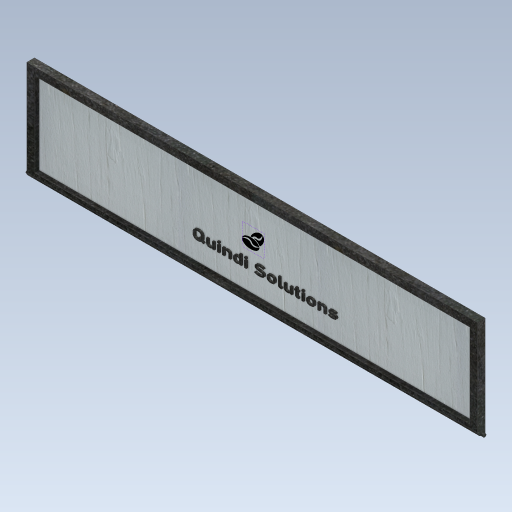
# Autodesk Inventor part: puerta
Saved by Autodesk Inventor 2023 (Build 270158000, 158)
## iProperties
Created: 2023-03-08
Part Number: puerta
Material: Steel
Document SubType Name: Modeling
Designer: santi
Density: 7.85 g/cm^3
Appearance: Plate
Author: santi
Autodesk Inventor part; units mm, degrees
ref_plane "YZ Plane" through (0, 0, 0) normal (1, 0, 0) x (0, 1, 0)
ref_plane "XZ Plane" through (0, 0, 0) normal (0, 1, 0) x (-1, 0, 0)
sketch "Sketch1" plane through (0, 0, 0) normal (0, 0, 1) x (1, 0, 0)
  line L0 (0, 0) -> (290, 0)
  line L1 (290, 0) -> (290, 64.12)
  line L2 (290, 64.12) -> (0, 64.12)
  line L3 (0, 64.12) -> (0, 0)
  line L4 (5, 59.12) -> (285, 59.12)
  line L5 (285, 59.12) -> (285, 5)
  line L6 (285, 5) -> (5, 5)
  line L7 (5, 5) -> (5, 59.12)
  dimension "d0" = 290
  dimension "d1" = 64.12
  dimension "d2" = 5
  constraints: 16 end point, 4 parallel, 2 perpendicular, 1 horizontal, 3 other
  measures "d0" distance of L2.end L1.end
  measures "d1" distance of L1.end L0.end
  measures "d2" distance between parallel lines of L2 L4
extrude "Extrusion1" add sketch "Sketch1" along normal blind 5
sketch "Sketch2" plane through (5, 5, 0) normal (1, 0, 0) x (0, 0, -1)
  line L0 (0, 54.12) -> (0, 0) projected
  line L1 (0, 54.12) -> (-5, 54.12) projected
  line L2 (0, 0) -> (-2, 0)
  line L3 (-2, 0) -> (-2, 54.12)
  line L4 (-2, 54.12) -> (0, 54.12)
  line L5 (0, 54.12) -> (0, 0)
  point P0 (0, -5)
  dimension "d5" = 2
  constraints: 8 end point, 2 parallel, 1 horizontal, 1 perpendicular, 1 point on line
  measures "d5" distance of L3.end L4.end
extrude "Extrusion2" add sketch "Sketch2" along normal up to surface (280 mm away)
sketch "Sketch3" plane through (0, 0, 0) normal (-1, 0, 0) x (0, 0, 1)
  circle A0 centre (2.5, 1) radius 1
  line L0 (5, 64.12) -> (5, 0) construction
  line L1 (0, 0) -> (5, 0) construction
  point P0 (2.5, 0)
  dimension "d8" = 2
  constraints: 1 centre point, 1 midpoint, 1 tangent, 1 vertical alignment
  measures "d8" diameter of A0
extrude "Extrusion3" add sketch "Sketch3" along normal blind 2 and the other way blind 2
ref_plane "Work Plane1" through (145, 0, 0) normal (1, 0, 0) x (0, 0, -1)
mirror "Mirror1" about plane through (145, 0, 0) normal (1, 0, 0) of "Extrusion3"
fillet "Fillet1" radius 2.7 1 edges at (145, 0, 5)
sketch "Sketch4" plane through (5, 5, 2) normal (0, 0, 1) x (1, 0, 0)
  line L0 (41.8121, 18.9) -> (199.4693, 18.9) construction
  line L1 (199.4693, 18.9) -> (199.4693, 1.1319) construction
  line L2 (199.4693, 1.1319) -> (41.8121, 1.1319) construction
  line L3 (41.8121, 1.1319) -> (41.8121, 18.9) construction
  line L4 (131.499, 39.7705) -> (150.9594, 39.7705) construction
  line L5 (150.9594, 39.7705) -> (150.9594, 20.3102) construction
  line L6 (150.9594, 20.3102) -> (131.499, 20.3102) construction
  line L7 (131.499, 20.3102) -> (131.499, 39.7705) construction
  spline S0 degree 2 poles (103.1114, 12.6741) (102.1443, 12.6741) (100.6936, 13.2282) (99.8927, 14.2457) (99.8927, 14.9207) knots 0 0 0 1 2 3 3 3
  line L8 (99.8927, 14.9207) -> (99.8927, 16.6484)
  spline S1 degree 2 poles (99.8927, 16.6484) (99.8927, 17.3284) (100.6936, 18.3409) (102.1443, 18.9) (103.1114, 18.9) knots 0 0 0 1 2 3 3 3
  spline S2 degree 2 poles (103.1114, 18.9) (104.0836, 18.9) (105.5292, 18.3409) (106.3302, 17.3284) (106.3302, 16.6484) knots 0 0 0 1 2 3 3 3
  line L9 (106.3302, 16.6484) -> (106.3302, 14.9207)
  spline S3 degree 2 poles (106.3302, 14.9207) (106.3302, 14.2457) (105.5292, 13.2282) (104.0836, 12.6741) (103.1114, 12.6741) knots 0 0 0 1 2 3 3 3
  spline S4 degree 2 poles (103.1114, 13.5153) (103.9728, 13.5153) (105.0155, 14.2709) (105.0155, 14.8904) knots 0 0 0 1 2 2 2
  line L10 (105.0155, 14.8904) -> (105.0155, 16.6786)
  spline S5 degree 2 poles (105.0155, 16.6786) (105.0155, 17.3032) (103.9728, 18.0538) (103.1114, 18.0538) knots 0 0 0 1 2 2 2
  spline S6 degree 2 poles (103.1114, 18.0538) (102.2551, 18.0538) (101.2124, 17.3032) (101.2124, 16.6786) knots 0 0 0 1 2 2 2
  line L11 (101.2124, 16.6786) -> (101.2124, 14.8904)
  spline S7 degree 2 poles (101.2124, 14.8904) (101.2124, 14.2709) (102.2551, 13.5153) (103.1114, 13.5153) knots 0 0 0 1 2 2 2
  line L12 (106.5065, 12.6338) -> (103.0913, 14.427)
  line L13 (103.0913, 14.427) -> (103.7612, 14.9912)
  line L14 (103.7612, 14.9912) -> (107.1714, 13.203)
  line L15 (107.1714, 13.203) -> (106.5065, 12.6338)
  line L16 (109.7151, 17.0917) -> (109.7151, 14.4421)
  spline S8 degree 2 poles (109.7151, 14.4421) (109.7151, 13.9837) (110.4153, 13.4851) (111.05, 13.4851) knots 0 0 0 1 2 2 2
  spline S9 degree 2 poles (111.05, 13.4851) (111.6847, 13.4851) (112.3697, 13.9334) (112.3697, 14.3414) knots 0 0 0 1 2 2 2
  line L17 (112.3697, 14.3414) -> (112.4604, 13.4297)
  spline S10 degree 2 poles (112.4604, 13.4297) (112.2841, 13.1375) (111.4026, 12.6741) (110.6923, 12.6741) knots 0 0 0 1 2 2 2
  spline S11 degree 2 poles (110.6923, 12.6741) (109.6093, 12.6741) (108.4306, 13.6009) (108.4306, 14.4421) knots 0 0 0 1 2 2 2
  line L18 (108.4306, 14.4421) -> (108.4306, 17.0917)
  line L19 (108.4306, 17.0917) -> (109.7151, 17.0917)
  line L20 (112.3697, 12.7345) -> (112.3697, 17.0917)
  line L21 (112.3697, 17.0917) -> (113.6491, 17.0917)
  line L22 (113.6491, 17.0917) -> (113.6491, 12.7345)
  line L23 (113.6491, 12.7345) -> (112.3697, 12.7345)
  line L24 (115.6036, 12.7345) -> (115.6036, 17.0917)
  line L25 (115.6036, 17.0917) -> (116.888, 17.0917)
  line L26 (116.888, 17.0917) -> (116.888, 12.7345)
  line L27 (116.888, 12.7345) -> (115.6036, 12.7345)
  line L28 (115.6036, 17.9782) -> (115.6036, 18.8345)
  line L29 (115.6036, 18.8345) -> (116.888, 18.8345)
  line L30 (116.888, 18.8345) -> (116.888, 17.9782)
  line L31 (116.888, 17.9782) -> (115.6036, 17.9782)
  line L32 (122.8017, 12.7345) -> (122.8017, 15.374)
  spline S12 degree 2 poles (122.8017, 15.374) (122.8017, 15.8374) (122.0914, 16.3411) (121.4366, 16.3411) knots 0 0 0 1 2 2 2
  spline S13 degree 2 poles (121.4366, 16.3411) (120.8069, 16.3411) (120.1219, 15.8928) (120.1219, 15.4899) knots 0 0 0 1 2 2 2
  line L33 (120.1219, 15.4899) -> (119.9909, 16.3311)
  spline S14 degree 2 poles (119.9909, 16.3311) (120.2932, 16.724) (121.2653, 17.1521) (121.8597, 17.1521) knots 0 0 0 1 2 2 2
  spline S15 degree 2 poles (121.8597, 17.1521) (122.9226, 17.1521) (124.0861, 16.2253) (124.0861, 15.379) knots 0 0 0 1 2 2 2
  line L34 (124.0861, 15.379) -> (124.0861, 12.7345)
  line L35 (124.0861, 12.7345) -> (122.8017, 12.7345)
  line L36 (118.8374, 12.7345) -> (118.8374, 17.0917)
  line L37 (118.8374, 17.0917) -> (120.1219, 17.0917)
  line L38 (120.1219, 17.0917) -> (120.1219, 12.7345)
  line L39 (120.1219, 12.7345) -> (118.8374, 12.7345)
  spline S16 degree 2 poles (128.1108, 12.659) (127.0278, 12.659) (125.8491, 13.5858) (125.8491, 14.4321) knots 0 0 0 1 2 2 2
  line L40 (125.8491, 14.4321) -> (125.8491, 15.3891)
  spline S17 degree 2 poles (125.8491, 15.3891) (125.8491, 16.2404) (127.0027, 17.1672) (128.0504, 17.1672) knots 0 0 0 1 2 2 2
  spline S18 degree 2 poles (128.0504, 17.1672) (128.6297, 17.1672) (129.5918, 16.7643) (129.8889, 16.3965) knots 0 0 0 1 2 2 2
  line L41 (129.8889, 16.3965) -> (129.7529, 15.51)
  spline S19 degree 2 poles (129.7529, 15.51) (129.7529, 15.7871) (129.4507, 16.1799) (128.8815, 16.3865) (128.4685, 16.3865) knots 0 0 0 1 2 3 3 3
  spline S20 degree 2 poles (128.4685, 16.3865) (127.8338, 16.3865) (127.1336, 15.8576) (127.1336, 15.379) knots 0 0 0 1 2 2 2
  line L42 (127.1336, 15.379) -> (127.1336, 14.4321)
  spline S21 degree 2 poles (127.1336, 14.4321) (127.1336, 13.9535) (127.8338, 13.4397) (128.4685, 13.4397) knots 0 0 0 1 2 2 2
  spline S22 degree 2 poles (128.4685, 13.4397) (128.8815, 13.4397) (129.4507, 13.6513) (129.7529, 14.0543) (129.7529, 14.3363) knots 0 0 0 1 2 3 3 3
  line L43 (129.7529, 14.3363) -> (129.8436, 13.4196)
  spline S23 degree 2 poles (129.8436, 13.4196) (129.6673, 13.1224) (128.806, 12.659) (128.1108, 12.659) knots 0 0 0 1 2 2 2
  line L44 (129.7529, 12.7345) -> (129.7529, 18.8345)
  line L45 (129.7529, 18.8345) -> (131.0374, 18.8345)
  line L46 (131.0374, 18.8345) -> (131.0374, 12.7345)
  line L47 (131.0374, 12.7345) -> (129.7529, 12.7345)
  line L48 (132.9918, 12.7345) -> (132.9918, 17.0917)
  line L49 (132.9918, 17.0917) -> (134.2763, 17.0917)
  line L50 (134.2763, 17.0917) -> (134.2763, 12.7345)
  line L51 (134.2763, 12.7345) -> (132.9918, 12.7345)
  line L52 (132.9918, 17.9782) -> (132.9918, 18.8345)
  line L53 (132.9918, 18.8345) -> (134.2763, 18.8345)
  line L54 (134.2763, 18.8345) -> (134.2763, 17.9782)
  line L55 (134.2763, 17.9782) -> (132.9918, 17.9782)
  spline S24 degree 2 poles (142.5624, 12.6741) (141.8975, 12.6741) (140.7188, 12.8403) (139.6913, 13.1728) (139.243, 13.4246) knots 0 0 0 1 2 3 3 3
  line L56 (139.243, 13.4246) -> (140.0439, 14.0795)
  spline S25 degree 2 poles (140.0439, 14.0795) (140.5677, 13.7772) (141.827, 13.475) (142.5624, 13.475) knots 0 0 0 1 2 2 2
  spline S26 degree 2 poles (142.5624, 13.475) (143.5598, 13.475) (144.6529, 13.9737) (144.6529, 14.4169) knots 0 0 0 1 2 2 2
  line L57 (144.6529, 14.4169) -> (144.6529, 14.422)
  spline S27 degree 2 poles (144.6529, 14.422) (144.6529, 14.7695) (144.0988, 15.1373) (143.1971, 15.3186) (142.6632, 15.379) knots 0 0 0 1 2 3 3 3
  spline S28 degree 2 poles (142.6632, 15.379) (142.1494, 15.4344) (141.0966, 15.5956) (140.2151, 15.9382) (139.6812, 16.5728) (139.6812, 17.1068) knots 0 0 0 1 2 3 4 4 4
  line L58 (139.6812, 17.1068) -> (139.6812, 17.1118)
  spline S29 degree 2 poles (139.6812, 17.1118) (139.6812, 17.9631) (141.3787, 18.9) (142.9302, 18.9) knots 0 0 0 1 2 2 2
  spline S30 degree 2 poles (142.9302, 18.9) (143.6656, 18.9) (145.076, 18.5827) (145.7409, 18.2603) knots 0 0 0 1 2 2 2
  line L59 (145.7409, 18.2603) -> (145.0105, 17.5803)
  spline S31 degree 2 poles (145.0105, 17.5803) (144.4917, 17.8422) (143.449, 18.0941) (142.9302, 18.0941) knots 0 0 0 1 2 2 2
  spline S32 degree 2 poles (142.9302, 18.0941) (141.9882, 18.0941) (140.9505, 17.5954) (140.9505, 17.137) knots 0 0 0 1 2 2 2
  line L60 (140.9505, 17.137) -> (140.9505, 17.132)
  spline S33 degree 2 poles (140.9505, 17.132) (140.9505, 16.7894) (141.555, 16.4268) (142.5322, 16.2555) (143.0913, 16.1799) knots 0 0 0 1 2 3 3 3
  spline S34 degree 2 poles (143.0913, 16.1799) (143.5951, 16.1145) (144.6025, 15.9231) (145.4286, 15.5654) (145.9273, 14.9458) (145.9273, 14.4472) knots 0 0 0 1 2 3 4 4 4
  line L61 (145.9273, 14.4472) -> (145.9273, 14.4371)
  spline S35 degree 2 poles (145.9273, 14.4371) (145.9273, 13.5959) (144.1643, 12.6741) (142.5624, 12.6741) knots 0 0 0 1 2 2 2
  spline S36 degree 2 poles (150.1283, 12.6741) (148.8438, 12.6741) (147.4334, 13.6664) (147.4334, 14.5681) knots 0 0 0 1 2 2 2
  line L62 (147.4334, 14.5681) -> (147.4334, 15.2783)
  spline S37 degree 2 poles (147.4334, 15.2783) (147.4334, 16.1699) (148.8438, 17.1521) (150.1283, 17.1521) knots 0 0 0 1 2 2 2
  spline S38 degree 2 poles (150.1283, 17.1521) (151.4127, 17.1521) (152.8231, 16.1699) (152.8231, 15.2783) knots 0 0 0 1 2 2 2
  line L63 (152.8231, 15.2783) -> (152.8231, 14.558)
  spline S39 degree 2 poles (152.8231, 14.558) (152.8231, 13.6563) (151.4127, 12.6741) (150.1283, 12.6741) knots 0 0 0 1 2 2 2
  spline S40 degree 2 poles (150.1283, 13.4851) (150.8032, 13.4851) (151.5387, 14.0492) (151.5387, 14.558) knots 0 0 0 1 2 2 2
  line L64 (151.5387, 14.558) -> (151.5387, 15.2783)
  spline S41 degree 2 poles (151.5387, 15.2783) (151.5387, 15.7871) (150.8032, 16.3411) (150.1283, 16.3411) knots 0 0 0 1 2 2 2
  spline S42 degree 2 poles (150.1283, 16.3411) (149.4633, 16.3411) (148.7178, 15.7871) (148.7178, 15.2783) knots 0 0 0 1 2 2 2
  line L65 (148.7178, 15.2783) -> (148.7178, 14.558)
  spline S43 degree 2 poles (148.7178, 14.558) (148.7178, 14.0492) (149.4633, 13.4851) (150.1283, 13.4851) knots 0 0 0 1 2 2 2
  line L66 (155.9361, 18.8345) -> (155.9361, 13.8578)
  spline S44 degree 2 poles (155.9361, 13.8578) (155.9361, 13.7017) (156.1426, 13.5254) (156.334, 13.5254) knots 0 0 0 1 2 2 2
  line L67 (156.334, 13.5254) -> (156.9385, 13.5254)
  line L68 (156.9385, 13.5254) -> (156.9385, 12.7144)
  line L69 (156.9385, 12.7144) -> (156.1829, 12.7144)
  spline S45 degree 2 poles (156.1829, 12.7144) (155.4576, 12.7144) (154.6516, 13.3188) (154.6516, 13.8679) knots 0 0 0 1 2 2 2
  line L70 (154.6516, 13.8679) -> (154.6516, 18.8345)
  line L71 (154.6516, 18.8345) -> (155.9361, 18.8345)
  line L72 (159.6686, 17.0917) -> (159.6686, 14.4421)
  spline S46 degree 2 poles (159.6686, 14.4421) (159.6686, 13.9837) (160.3688, 13.4851) (161.0035, 13.4851) knots 0 0 0 1 2 2 2
  spline S47 degree 2 poles (161.0035, 13.4851) (161.6382, 13.4851) (162.3232, 13.9334) (162.3232, 14.3414) knots 0 0 0 1 2 2 2
  line L73 (162.3232, 14.3414) -> (162.4139, 13.4297)
  spline S48 degree 2 poles (162.4139, 13.4297) (162.2376, 13.1375) (161.3561, 12.6741) (160.6458, 12.6741) knots 0 0 0 1 2 2 2
  spline S49 degree 2 poles (160.6458, 12.6741) (159.5629, 12.6741) (158.3842, 13.6009) (158.3842, 14.4421) knots 0 0 0 1 2 2 2
  line L74 (158.3842, 14.4421) -> (158.3842, 17.0917)
  line L75 (158.3842, 17.0917) -> (159.6686, 17.0917)
  line L76 (162.3232, 12.7345) -> (162.3232, 17.0917)
  line L77 (162.3232, 17.0917) -> (163.6027, 17.0917)
  line L78 (163.6027, 17.0917) -> (163.6027, 12.7345)
  line L79 (163.6027, 12.7345) -> (162.3232, 12.7345)
  spline S50 degree 2 poles (167.2546, 12.7144) (166.4486, 12.7144) (165.7283, 13.3088) (165.7283, 13.8679) knots 0 0 0 1 2 2 2
  line L80 (165.7283, 13.8679) -> (165.7283, 18.356)
  line L81 (165.7283, 18.356) -> (167.0128, 18.356)
  line L82 (167.0128, 18.356) -> (167.0128, 13.8578)
  spline S51 degree 2 poles (167.0128, 13.8578) (167.0128, 13.7017) (167.1992, 13.5254) (167.3805, 13.5254) knots 0 0 0 1 2 2 2
  line L83 (167.3805, 13.5254) -> (168.0001, 13.5254)
  line L84 (168.0001, 13.5254) -> (168.0001, 12.7144)
  line L85 (168.0001, 12.7144) -> (167.2546, 12.7144)
  line L86 (165.0534, 16.316) -> (165.0534, 17.0917)
  line L87 (165.0534, 17.0917) -> (168.0001, 17.0917)
  line L88 (168.0001, 17.0917) -> (168.0001, 16.316)
  line L89 (168.0001, 16.316) -> (165.0534, 16.316)
  line L90 (169.7631, 12.7345) -> (169.7631, 17.0917)
  line L91 (169.7631, 17.0917) -> (171.0476, 17.0917)
  line L92 (171.0476, 17.0917) -> (171.0476, 12.7345)
  line L93 (171.0476, 12.7345) -> (169.7631, 12.7345)
  line L94 (169.7631, 17.9782) -> (169.7631, 18.8345)
  line L95 (169.7631, 18.8345) -> (171.0476, 18.8345)
  line L96 (171.0476, 18.8345) -> (171.0476, 17.9782)
  line L97 (171.0476, 17.9782) -> (169.7631, 17.9782)
  spline S52 degree 2 poles (175.5004, 12.6741) (174.2159, 12.6741) (172.8055, 13.6664) (172.8055, 14.5681) knots 0 0 0 1 2 2 2
  line L98 (172.8055, 14.5681) -> (172.8055, 15.2783)
  spline S53 degree 2 poles (172.8055, 15.2783) (172.8055, 16.1699) (174.2159, 17.1521) (175.5004, 17.1521) knots 0 0 0 1 2 2 2
  spline S54 degree 2 poles (175.5004, 17.1521) (176.7849, 17.1521) (178.1953, 16.1699) (178.1953, 15.2783) knots 0 0 0 1 2 2 2
  line L99 (178.1953, 15.2783) -> (178.1953, 14.558)
  spline S55 degree 2 poles (178.1953, 14.558) (178.1953, 13.6563) (176.7849, 12.6741) (175.5004, 12.6741) knots 0 0 0 1 2 2 2
  spline S56 degree 2 poles (175.5004, 13.4851) (176.1754, 13.4851) (176.9108, 14.0492) (176.9108, 14.558) knots 0 0 0 1 2 2 2
  line L100 (176.9108, 14.558) -> (176.9108, 15.2783)
  spline S57 degree 2 poles (176.9108, 15.2783) (176.9108, 15.7871) (176.1754, 16.3411) (175.5004, 16.3411) knots 0 0 0 1 2 2 2
  spline S58 degree 2 poles (175.5004, 16.3411) (174.8355, 16.3411) (174.09, 15.7871) (174.09, 15.2783) knots 0 0 0 1 2 2 2
  line L101 (174.09, 15.2783) -> (174.09, 14.558)
  spline S59 degree 2 poles (174.09, 14.558) (174.09, 14.0492) (174.8355, 13.4851) (175.5004, 13.4851) knots 0 0 0 1 2 2 2
  line L102 (183.988, 12.7345) -> (183.988, 15.374)
  spline S60 degree 2 poles (183.988, 15.374) (183.988, 15.8374) (183.2778, 16.3411) (182.623, 16.3411) knots 0 0 0 1 2 2 2
  spline S61 degree 2 poles (182.623, 16.3411) (181.9933, 16.3411) (181.3083, 15.8928) (181.3083, 15.4899) knots 0 0 0 1 2 2 2
  line L103 (181.3083, 15.4899) -> (181.1773, 16.3311)
  spline S62 degree 2 poles (181.1773, 16.3311) (181.4795, 16.724) (182.4517, 17.1521) (183.0461, 17.1521) knots 0 0 0 1 2 2 2
  spline S63 degree 2 poles (183.0461, 17.1521) (184.1089, 17.1521) (185.2725, 16.2253) (185.2725, 15.379) knots 0 0 0 1 2 2 2
  line L104 (185.2725, 15.379) -> (185.2725, 12.7345)
  line L105 (185.2725, 12.7345) -> (183.988, 12.7345)
  line L106 (180.0238, 12.7345) -> (180.0238, 17.0917)
  line L107 (180.0238, 17.0917) -> (181.3083, 17.0917)
  line L108 (181.3083, 17.0917) -> (181.3083, 12.7345)
  line L109 (181.3083, 12.7345) -> (180.0238, 12.7345)
  spline S64 degree 2 poles (189.539, 12.6741) (188.6676, 12.6741) (187.2521, 13.0116) (186.693, 13.3491) knots 0 0 0 1 2 2 2
  line L110 (186.693, 13.3491) -> (187.4536, 13.9787)
  spline S65 degree 2 poles (187.4536, 13.9787) (187.9875, 13.7067) (189.0252, 13.4397) (189.539, 13.4397) knots 0 0 0 1 2 2 2
  spline S66 degree 2 poles (189.539, 13.4397) (190.2996, 13.4397) (191.0602, 13.752) (191.0602, 14.0694) knots 0 0 0 1 2 2 2
  spline S67 degree 2 poles (191.0602, 14.0694) (191.0602, 14.3112) (190.5515, 14.5126) (189.7254, 14.5781) (189.2519, 14.5983) knots 0 0 0 1 2 3 3 3
  spline S68 degree 2 poles (189.2519, 14.5983) (188.859, 14.6184) (188.0782, 14.7091) (187.4335, 14.9358) (187.0506, 15.3891) (187.0506, 15.7719) knots 0 0 0 1 2 3 4 4 4
  spline S69 degree 2 poles (187.0506, 15.7719) (187.0506, 16.4671) (188.32, 17.1521) (189.5793, 17.1521) knots 0 0 0 1 2 2 2
  spline S70 degree 2 poles (189.5793, 17.1521) (190.35, 17.1521) (191.6697, 16.8751) (192.249, 16.593) knots 0 0 0 1 2 2 2
  line L111 (192.249, 16.593) -> (191.4783, 15.9634)
  spline S71 degree 2 poles (191.4783, 15.9634) (190.9847, 16.1749) (190.0326, 16.3865) (189.5793, 16.3865) knots 0 0 0 1 2 2 2
  spline S72 degree 2 poles (189.5793, 16.3865) (188.9245, 16.3865) (188.2696, 16.0893) (188.2696, 15.7871) knots 0 0 0 1 2 2 2
  spline S73 degree 2 poles (188.2696, 15.7871) (188.2696, 15.5906) (188.723, 15.4193) (189.4685, 15.369) (189.8966, 15.3488) knots 0 0 0 1 2 3 3 3
  spline S74 degree 2 poles (189.8966, 15.3488) (190.3046, 15.3337) (191.1408, 15.243) (191.846, 14.9912) (192.2742, 14.4975) (192.2742, 14.0694) knots 0 0 0 1 2 3 4 4 4
  spline S75 degree 2 poles (192.2742, 14.0694) (192.2742, 13.3692) (190.9091, 12.6741) (189.539, 12.6741) knots 0 0 0 1 2 2 2
  point P0 (-5, -5)
  constraints: 4 other
emboss "Emboss1" sketch "Sketch4" operation add depth 1 direction (0, 0, -1) contours S0 L8 S1 S2 L9 S3 L14 S4 L10 S5 S6 L11 S7 L12 | L12 S4 L14 S3 | S3 L14 L15 L12 | L12 L13 L14 S4 | L16 S8 S9 L20 S10 S11 L18 L19 | L20 L21 L22 L23 S10 L17 | L17 S10 L20 | L24 L25 L26 L27 | L28 L29 L30 L31 | L32 S12 S13 L38 S14 S15 L34 L35 | L38 L39 L36 L37 S14 L33 | L33 S14 L38 | S16 L40 S17 S18 L44 S19 S20 L42 S21 S22 S23 | L44 L43 S23 | S23 L43 L44 L41 S18 L45 L46 L47 | L44 S18 L41 | L48 L49 L50 L51 | L52 L53 L54 L55 | S24 L56 S25 S26 L57 S27 S28 L58 S29 S30 L59 S31 S32 L60 S33 S34 L61 S35 | S36 L62 S37 S38 L63 S39 | L66 S44 L67 L68 L69 S45 L70 L71 | L72 S46 S47 L76 S48 S49 L74 L75 | L76 L77 L78 L79 S48 L73 | L73 S48 L76 | S50 L80 L89 L82 S51 L83 L84 L85 | L89 L86 L87 L80 | L80 L87 L82 L89 | L80 L81 L82 L87 | L82 L87 L88 L89 | L90 L91 L92 L93 | L94 L95 L96 L97 | S52 L98 S53 S54 L99 S55 | L102 S60 S61 L108 S62 S63 L104 L105 | L108 L109 L106 L107 S62 L103 | L103 S62 L108 | S64 L110 S65 S66 S67 S68 S69 S70 L111 S71 S72 S73 S74 S75
sketch "Sketch5" plane through (5, 5, 2) normal (0, 0, 1) x (1, 0, 0)
  line L0 (130.5228, 37.0857) -> (144.6811, 37.0857) construction
  line L1 (144.6811, 37.0857) -> (144.6811, 22.9274) construction
  line L2 (144.6811, 22.9274) -> (130.5228, 22.9274) construction
  line L3 (130.5228, 22.9274) -> (130.5228, 37.0857) construction
  point P0 (-5, -5)
  constraints: 2 other
body "Solid1"
